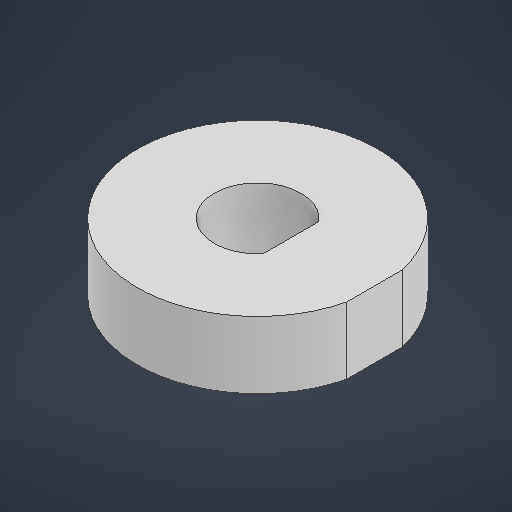
# Autodesk Inventor part: tronco_ruota_2
Saved by Autodesk Inventor 2027 (Build 310192060, 192F)
## iProperties
Created: 2026-07-02
Part Number: tronco_ruota_2
Material: Generic
Document SubType Name: Modeling
Designer: loren
Density: 1 g/cm^3
Appearance: Default
Author: loren
Autodesk Inventor part; units mm, degrees
ref_plane "YZ Plane" through (0, 0, 0) normal (1, 0, 0) x (0, 1, 0)
ref_plane "XZ Plane" through (0, 0, 0) normal (0, 1, 0) x (-1, 0, 0)
ref_plane "XY Plane" through (0, 0, 0) normal (0, 0, 1) x (1, 0, 0)
sketch "Sketch1" plane through (0, 0, 0) normal (0, 1, 0) x (-1, 0, 0)
  line L0 (-1.0005, 0.83) -> (-1.0005, -0.83)
  arc A0 (-1.0005, -0.83) -> (-1.0005, 0.83) centre (0, 0) ccw
  line L1 (-3.5, 0.83) -> (-3.5, -0.83)
  arc A1 (-3.5, -0.83) -> (-3.5, 0.83) centre (0, 0) ccw
  point P0 (0, 0)
  dimension "d0" = 1.66
  dimension "d1" = 1.3
  constraints: 4 end point, 4 point on circle, 2 centre point, 2 vertical, 1 coincident
  measures "d0" distance of L0.start L0.end
  measures "d1" radius of A0
extrude "Extrusion1" add sketch "Sketch1" along normal blind 2
body "Solid1"
